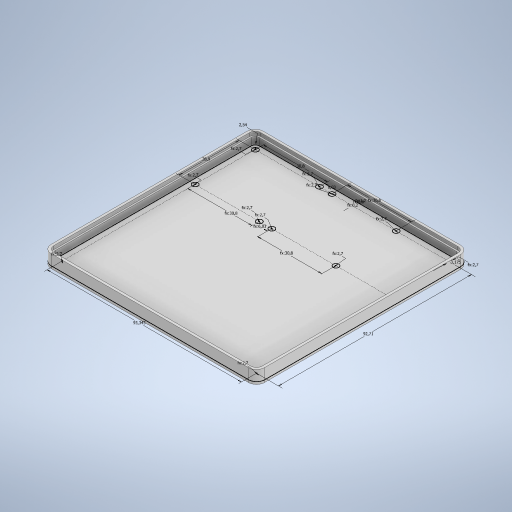
# Autodesk Inventor part: Housing_Bottom
Saved by Autodesk Inventor 2023 (Build 270158000, 158)
## iProperties
Created: 2023-02-18
Part Number: Housing_Bottom
Material: Generisch
Document SubType Name: Modeling
Designer: dvd62
Density: 1 g/cm^3
Appearance: Vorgabe
Author: dvd62
Autodesk Inventor part; units mm, degrees
ref_plane "YZ Plane" through (0, 0, 0) normal (1, 0, 0) x (0, 1, 0)
ref_plane "XZ Plane" through (0, 0, 0) normal (0, 1, 0) x (-1, 0, 0)
ref_plane "XY Plane" through (0, 0, 0) normal (0, 0, 1) x (1, 0, 0)
sketch "Skizze1" plane through (0, 0, 0) normal (0, 1, 0) x (-1, 0, 0)
  circle A0 centre (0, 0) radius 1.35
  line L0 (0, 0) -> (-93.345, 0) construction
  line L1 (-93.345, 0) -> (-93.345, -92.71) construction
  line L2 (-93.345, -92.71) -> (0, -92.71) construction
  line L3 (0, -92.71) -> (0, 0) construction
  circle A1 centre (0, -92.71) radius 1.35
  circle A2 centre (-93.345, -92.71) radius 1.35
  circle A3 centre (-93.345, 0) radius 1.35
  circle A4 centre (-30.8, -92.71) radius 1.35
  circle A5 centre (-36.83, -92.71) radius 1.35
  circle A6 centre (-67.63, -92.71) radius 1.35
  line L4 (0, -63.81) -> (-93.345, -63.81) construction
  circle A7 centre (0, -63.81) radius 1.35
  circle A8 centre (-30.8, -63.81) radius 1.35
  circle A9 centre (-36.83, -63.81) radius 1.35
  circle A10 centre (-67.63, -63.81) radius 1.35
  line L5 (0.635, -95.885) -> (-93.98, -95.885) construction
  line L6 (-96.52, -93.345) -> (-96.52, 0.635) construction
  line L7 (-93.98, 3.175) -> (0.635, 3.175) construction
  line L8 (3.175, 0.635) -> (3.175, -93.345) construction
  arc A11 (0.635, -95.885) -> (3.175, -93.345) centre (0.635, -93.345) ccw construction
  arc A12 (-96.52, -93.345) -> (-93.98, -95.885) centre (-93.98, -93.345) ccw construction
  arc A13 (-93.98, 3.175) -> (-96.52, 0.635) centre (-93.98, 0.635) ccw construction
  arc A14 (3.175, 0.635) -> (0.635, 3.175) centre (0.635, 0.635) ccw construction
  line L9 (-93.98, -96.085) -> (0.635, -96.085)
  arc A15 (0.635, -96.085) -> (3.375, -93.345) centre (0.635, -93.345) ccw
  line L10 (3.375, -93.345) -> (3.375, 0.635)
  arc A16 (3.375, 0.635) -> (0.635, 3.375) centre (0.635, 0.635) ccw
  line L11 (0.635, 3.375) -> (-93.98, 3.375)
  arc A17 (-93.98, 3.375) -> (-96.72, 0.635) centre (-93.98, 0.635) ccw
  line L12 (-96.72, 0.635) -> (-96.72, -93.345)
  arc A18 (-96.72, -93.345) -> (-93.98, -96.085) centre (-93.98, -93.345) ccw
  line L13 (0.635, -97.285) -> (-93.98, -97.285)
  arc A19 (-97.92, -93.345) -> (-93.98, -97.285) centre (-93.98, -93.345) ccw
  line L14 (-97.92, -93.345) -> (-97.92, 0.635)
  arc A20 (-93.98, 4.575) -> (-97.92, 0.635) centre (-93.98, 0.635) ccw
  line L15 (-93.98, 4.575) -> (0.635, 4.575)
  arc A21 (4.575, 0.635) -> (0.635, 4.575) centre (0.635, 0.635) ccw
  line L16 (4.575, 0.635) -> (4.575, -93.345)
  arc A22 (0.635, -97.285) -> (4.575, -93.345) centre (0.635, -93.345) ccw
  line L17 (0.635, -95.285) -> (-93.98, -95.285)
  arc A23 (-95.92, -93.345) -> (-93.98, -95.285) centre (-93.98, -93.345) ccw
  line L18 (-95.92, -93.345) -> (-95.92, 0.635)
  arc A24 (-93.98, 2.575) -> (-95.92, 0.635) centre (-93.98, 0.635) ccw
  line L19 (-93.98, 2.575) -> (0.635, 2.575)
  arc A25 (2.575, 0.635) -> (0.635, 2.575) centre (0.635, 0.635) ccw
  line L20 (2.575, 0.635) -> (2.575, -93.345)
  arc A26 (0.635, -95.285) -> (2.575, -93.345) centre (0.635, -93.345) ccw
  dimension "d0" = 2.7
  dimension "d1" = 2.7
  dimension "d2" = 2.7
  dimension "d3" = 2.7
  dimension "d4" = 93.345
  dimension "d5" = 92.71
  dimension "d6" = 2.7
  dimension "d7" = 2.7
  dimension "d8" = 2.7
  dimension "d10" = 2.7
  dimension "d11" = 2.7
  dimension "d12" = 2.7
  dimension "d13" = 2.7
  dimension "d14" = 28.9
  dimension "d15" = 30.8
  dimension "d16" = 6.03
  dimension "d17" = 30.8
  dimension "d18" = 30.8
  dimension "d19" = 6.03
  dimension "d20" = 30.8
  dimension "d21" = 3.175
  dimension "d22" = 2.54
  dimension "d23" = 0.2
  dimension "d24" = 1.2
  dimension "d29" = 0.8
  constraints: 42 end point, 32 point on circle, 27 centre point, 10 parallel, 8 point on line, 8 tangent, 6 perpendicular, 5 coincident, 3 equal radius, 1 horizontal, 24 other
  measures "d0" diameter of A0
  measures "d1" diameter of A1
  measures "d2" diameter of A2
  measures "d3" diameter of A3
  measures "d4" distance of L0.start L0.end
  measures "d5" distance of L0.end L1.end
  measures "d6" diameter of A4
  measures "d7" diameter of A5
  measures "d8" diameter of A6
  measures "d10" diameter of A7
  measures "d11" diameter of A8
  measures "d12" diameter of A9
  measures "d13" diameter of A10
  measures "d14" distance between parallel lines of L2 L4
  measures "d15" distance of A4.centre A1.centre
  measures "d16" distance of A5.centre A4.centre
  measures "d17" distance of A6.centre A5.centre
  measures "d18" distance of A8.centre A7.centre
  measures "d19" distance of A8.centre A9.centre
  measures "d20" distance of A9.centre A10.centre
  measures "d21" distance between parallel lines of L5 L2
  measures "d22" radius of A11
  measures "d23" distance between parallel lines of L5 L9
  measures "d24" distance between parallel lines of L9 L13
  measures "d29" distance between parallel lines of L9 L17
extrude "Extrusion1" add sketch "Skizze1" against normal blind 1.2 contours A0 | A1 | A2 | A3 | A4 | A5 | A6 | A7 | A8 | A9 | A10 | A18 L12 A17 L11 A16 L10 A15 L9 | L13 A19 L14 A20 L15 A21 L16 A22 | L17 A23 L18 A24 L19 A25 L20 A26
extrude "Extrusion2" add sketch "Skizze1" along normal blind 5 contours L13 A19 L14 A20 L15 A21 L16 A22
extrude "Extrusion3" add sketch "Skizze1" along normal blind 3.4 contours A18 L12 A17 L11 A16 L10 A15 L9
equation "\"d0\" = holeDim"
equation "\"d1\" = holeDim"
equation "\"d2\" = holeDim"
equation "\"d3\" = holeDim"
equation "\"d6\" = holeDim"
equation "\"d7\" = holeDim"
equation "\"d8\" = holeDim"
equation "\"d10\" = holeDim"
equation "\"d11\" = holeDim"
equation "\"d12\" = holeDim"
equation "\"d13\" = holeDim"
equation "\"d17\" = d15"
equation "\"d18\" = d15"
equation "\"d19\" = d16"
equation "\"d20\" = d15"
equation "\"d23\" = airGabWall"
equation "\"d24\" = topWallThick"
equation "\"d29\" = baseWallThick"
equation "\"d25\" = baseThick"
equation "\"d27\" = heightWall"
equation "\"d30\" = baseHeightWall"
equation "\"holeDim\" = 2.7"
equation "\"topWallThick\" = 1.2"
equation "\"airGabWall\" = 0.2"
equation "\"baseThick\" = 1.2"
equation "\"heightWall\" = 5"
equation "\"baseWallThick\" = 0.8"
equation "\"pcbThick\" = 1.6"
equation "\"baseHeightWall\" = heightWall - pcbThick"
